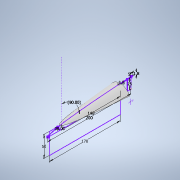
# Autodesk Inventor part: nose-toppart1
Saved by Autodesk Inventor 2020.3 (Build 243373000, 373)
## iProperties
Created: 2021-03-10
Part Number: nose-toppart1
Material: Generic
Document SubType Name: Modeling
Designer: 0x6f736f646f
Density: 1 g/cm^3
Appearance: Default
Author: 0x6f736f646f
Autodesk Inventor part; units mm, degrees
ref_plane "YZ Plane" through (0, 0, 0) normal (1, 0, 0) x (0, 1, 0)
ref_plane "XZ Plane" through (0, 0, 0) normal (0, 1, 0) x (-1, 0, 0)
ref_plane "XY Plane" through (0, 0, 0) normal (0, 0, 1) x (1, 0, 0)
sketch "Sketch1" plane through (0, 0, 0) normal (1, 0, 0) x (0, 1, 0)
  line L0 (0, 0) -> (25, 0)
  line L1 (25, 0) -> (25, -5)
  line L2 (25, -5) -> (26.8, -5)
  line L3 (26.8, -5) -> (26.8, 0)
  line L4 (0, 0) -> (0, 200)
  spline S0 degree 2 poles (26.8, 0) (13.4, 200) (0, 200) knots 0 0 0 1 1 1
  line L5 (1.9566, 200) -> (-1.9566, 200) construction
  arc A0 (1.1799, 199.5579) -> (-1.1799, 199.5579) centre (0, 198.2044) ccw construction
  line L6 (0, 160.0002) -> (11.7504, 160.0002) construction
  line L7 (0, 161.8) -> (13.7857, 161.8) construction
  line L8 (0, 10) -> (26.1214, 10)
  line L9 (0, 8.2) -> (24.4774, 8.2)
  line L10 (24.5307, 7.3724) -> (24.4241, 9.0276) construction
  arc A1 (24.52, 7.5379) -> (24.4347, 8.8621) centre (-5899.3235, -373.3767) ccw construction
  spline S1 degree 2 poles (25, 0) (24.7387, 4.1433) (24.4774, 8.2) knots 0 0 0 1 1 1
  line L11 (10.1029, 165.8331) -> (10.1029, 25.8331)
  line L12 (10.1029, 165.8331) -> (150.1029, 165.8331) construction
  line L13 (10.1029, 25.8331) -> (25.0094, 25.8331)
  line L14 (0, 170) -> (9.3945, 175.4239)
  line L15 (0, 170) -> (11.3645, 170) construction
  line L16 (0, 171.8) -> (8.2591, 176.5684)
  line L17 (0, 171.8) -> (0, 170)
  line L18 (10.1897, 166.1244) -> (6.942, 183.7666) construction
  arc A2 (9.7692, 167.8737) -> (7.172, 181.9822) centre (-252.6717, 126.854) ccw construction
  line L19 (9.1499, 171.9152) -> (7.373, 181.2243) construction
  arc A3 (8.9426, 172.8409) -> (7.5213, 180.2873) centre (-226.6717, 131.7265) ccw construction
  spline S2 degree 2 poles (24.4774, 8.2) (16.522, 131.7266) (8.5658, 174.9455) knots 0 0 0 1 1 1
  spline S3 degree 2 poles (8.2614, 176.5697) (4.1308, 198.2099) (0, 198.2044) knots 0 0 0 1 1 1
  line L20 (8.2591, 176.5684) -> (8.2614, 176.5697)
  line L21 (10.1029, 165.8331) -> (10.1029, 171.5783)
  line L22 (10.1029, 165.8331) -> (10.1029, 177.6329)
  line L23 (0, 0) -> (25, 0)
  line L24 (25, 0) -> (25, -5)
  line L25 (25, -5) -> (26.8, -5)
  line L26 (26.8, -5) -> (26.8, 0)
  line L27 (0, 0) -> (0, 200)
  spline S4 degree 2 poles (26.8, 0) (13.4, 200) (0, 200) knots 0 0 0 1 1 1
  line L28 (1.9566, 200) -> (-1.9566, 200) construction
  arc A4 (1.1799, 199.5579) -> (-1.1799, 199.5579) centre (0, 198.2044) ccw construction
  line L29 (0, 160.0002) -> (11.7504, 160.0002) construction
  line L30 (0, 161.8) -> (13.7857, 161.8) construction
  line L31 (24.5307, 7.3724) -> (24.4241, 9.0276) construction
  arc A5 (24.52, 7.5379) -> (24.4347, 8.8621) centre (-5899.3217, -373.3766) ccw construction
  spline S5 degree 2 poles (25, 0) (24.7387, 4.1433) (24.4774, 8.2) knots 0 0 0 1 1 1
  line L32 (10.1029, 165.8331) -> (10.1029, 25.8331)
  line L33 (10.1029, 165.8331) -> (150.1029, 165.8331) construction
  line L34 (10.1029, 25.8331) -> (25.0094, 25.8331)
  line L35 (0, 170) -> (9.3945, 175.4239)
  line L36 (0, 170) -> (11.3645, 170) construction
  line L37 (0, 171.8) -> (8.2591, 176.5684)
  line L38 (0, 171.8) -> (0, 170)
  line L39 (10.1897, 166.1244) -> (6.942, 183.7666) construction
  arc A6 (9.7692, 167.8737) -> (7.172, 181.9822) centre (-252.6717, 126.854) ccw construction
  line L40 (9.1499, 171.9152) -> (7.373, 181.2243) construction
  arc A7 (8.9426, 172.8409) -> (7.5213, 180.2873) centre (-226.6717, 131.7265) ccw construction
  spline S6 degree 2 poles (24.4774, 8.2) (16.522, 131.7266) (8.5658, 174.9455) knots 0 0 0 1 1 1
  spline S7 degree 2 poles (8.2614, 176.5697) (4.1308, 198.2099) (0, 198.2044) knots 0 0 0 1 1 1
  line L41 (8.2591, 176.5684) -> (8.2614, 176.5697)
  line L42 (0, 24.0331) -> (23.4355, 24.0331)
  line L43 (0, 22.2331) -> (23.5563, 22.2331)
  line L44 (10.1029, 25.8331) -> (0, 25.8331)
  line L45 (10.1029, 25.8331) -> (-39.8971, 25.8331)
  line L46 (-39.8971, 25.8331) -> (-39.8971, 195.8331)
  line L47 (-39.8971, 195.8331) -> (10.1029, 195.8331)
  line L48 (10.1029, 195.8331) -> (10.1029, 25.8331)
  point P0 (0, 0)
  point P1 (-25, 0)
  point P2 (-26.8, 0)
  point P3 (0, 198.2)
  point P4 (24.3612, 10)
  point P5 (24.3612, 10)
  point P6 (10.1029, 165.8469)
  point P7 (23.3141, 25.8331)
  point P8 (-25, 0)
  point P9 (-26.8, 0)
  point P10 (0, 198.2)
  point P11 (0, 10)
  point P12 (0, 8.2)
  point P13 (24.3612, 10)
  point P14 (23.3141, 25.8331)
  point P15 (0, 25.8331)
  point P16 (10.1029, 25.8331)
  point P17 (0, 25.8331)
  dimension "d0" = 25
  dimension "d1" = 5
  dimension "d2" = 1.8
  dimension "d3" = 200
  dimension "d4" = 140
  dimension "d5" = 90
  dimension "d6" = 30
  dimension "d8" = 25
  dimension "d9" = 5
  dimension "d10" = 1.8
  dimension "d11" = 200
  dimension "d12" = 140
  dimension "d13" = 90
  dimension "d14" = 30
  dimension "d15" = 1.8
  dimension "d16" = 1.8
  dimension "d19" = 50
  dimension "d20" = 170
  constraints: 94 end point, 16 midpoint, 15 horizontal, 11 perpendicular, 8 centre point, 8 point on circle, 6 vertical, 5 parallel, 5 point on line, 63 other
  measures "d0" distance of L0.start L0.end
  measures "d1" distance of L0.end L1.end
  measures "d2" distance of L1.end L2.end
  measures "d3" distance of point (0, 200) L0.start
  measures "d4" distance of L11.start L11.end
  measures "d5" angle of L11 L12
  measures "d6" angle of L15 L14
  measures "d8" distance of L23.start L23.end
  measures "d9" distance of L23.end L24.end
  measures "d10" distance of L24.end L25.end
  measures "d11" distance of point (0, 200) L23.start
  measures "d12" distance of L32.start L32.end
  measures "d13" angle of L32 L33
  measures "d14" angle of L36 L35
  measures "d15" distance between parallel lines of L42 L34
  measures "d16" distance between parallel lines of L43 L42
  measures "d19" distance of L46.end L47.end
  measures "d20" distance of L45.end L46.end
revolve "Revolution1" add sketch "Sketch1" angle 210 mid plane about axis through (0, 0, 0) along (0, 0, 1) contours L13 S2 L21 S0
extrude "Extrusion2" cut sketch "Sketch1" along normal mid plane 50 contours L45 L46 L47 L4 | L4 L14 S2 L11 L44 | L21 S2 L14 S0 | S0 L47 L48 L22 | L4 L16 L20 S3 L47 S0 L14 | L4 L47 S3 L20 L16
body "Solid1"
